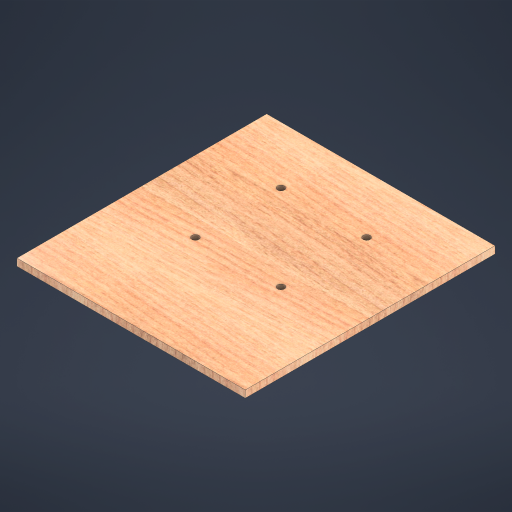
# Autodesk Inventor part: deska
Saved by Autodesk Inventor 2023 (Build 270158000, 158)
## iProperties
Created: 2022-10-19
Part Number: deska
Material: Dřevo (Bříza)
Document SubType Name: Modeling
Designer: zak
Density: 0.55 g/cm^3
Appearance: Bříza – přírodní leštěná
Mass: 614.21 g
Surface Area: 2382.55 cm^2
Volume: 1116.75 cm^3
Author: zak
Autodesk Inventor part; units mm, degrees
ref_plane "YZ Plane" through (0, 0, 0) normal (1, 0, 0) x (0, 1, 0)
ref_plane "XZ Plane" through (0, 0, 0) normal (0, 1, 0) x (-1, 0, 0)
ref_plane "XY Plane" through (0, 0, 0) normal (0, 0, 1) x (1, 0, 0)
sketch "Náčrt1" plane through (0, 0, 0) normal (0, 1, 0) x (-1, 0, 0)
  line L0 (160, 175) -> (-160, 175)
  line L1 (-160, 175) -> (-160, -175)
  line L2 (-160, -175) -> (160, -175)
  line L3 (160, -175) -> (160, 175)
  line L4 (160, 175) -> (-160, -175) construction
  line L5 (-160, 175) -> (160, -175) construction
  point P0 (0, 0)
  dimension "d0" = 320
  dimension "d1" = 350
  constraints: 12 end point, 2 midpoint, 2 parallel, 1 horizontal, 1 perpendicular
  measures "d0" distance of L2.end L1.end
  measures "d1" distance of L1.end L0.end
extrude "Vysunutí1" add sketch "Náčrt1" along normal blind 10
sketch "Náčrt3" plane through (0, 0, 0) normal (0, -1, 0) x (1, 0, 0)
  line L0 (160, -175) -> (-160, -175) projected
  line L1 (160, 175) -> (160, -175) projected
  point P0 (0, 0)
  point P1 (60, -95)
  point P2 (60, 25)
  point P3 (-60, 25)
  point P4 (-60, -95)
  dimension "d14" = 120
  dimension "d15" = 120
  dimension "d16" = 80
  dimension "d17" = 100
  constraints: 2 horizontal alignment, 2 vertical alignment
  measures "d14" distance of point (-60, -95) point (60, -95)
  measures "d15" distance of point (60, -95) point (60, 25)
  measures "d16" distance from line of L0 point (60, -95)
  measures "d17" distance from line of L1 point (60, -95)
hole "Díra1" at (60, 0, -95) at (60, 0, 25) at (-60, 0, 25) at (-60, 0, -95) direction (0, 1, 0) diameter 10 end through all
sketch "Náčrt4" plane through (0, 0, 0) normal (0, -1, 0) x (1, 0, 0)
  line L0 (-160, 175) -> (160, 175) projected
  line L1 (-160, -175) -> (-160, 175) projected
  line L2 (160, 175) -> (160, -175) projected
  line L3 (160, -175) -> (-160, -175) projected
  point P0 (0, 0)
  point P1 (-140, 155)
  point P2 (140, 155)
  point P3 (-140, -155)
  point P4 (140, -155)
  dimension "d25" = 20
  dimension "d26" = 20
  dimension "d27" = 20
  dimension "d28" = 20
  constraints: 2 horizontal alignment, 2 vertical alignment
  measures "d25" distance from line of point (-140, 155) L0
  measures "d26" distance from line of point (-140, 155) L1
  measures "d27" distance from line of L2 point (140, 155)
  measures "d28" distance from line of L3 point (140, -155)
hole "Díra2" at (-140, 0, 155) at (140, 0, 155) at (-140, 0, -155) at (140, 0, -155) direction (0, 1, 0) diameter 2 depth 9
